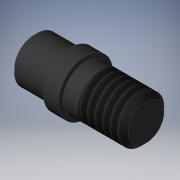
# Autodesk Inventor part: NTBG6-4_a
Saved by Autodesk Inventor 2019 (Build 230136000, 136)
## iProperties
Created: 2023-12-09
Part Number: NTBG6-4_a
Material: Generic
Catalog Web Link: www.cadenas.de
Description: NTBG, NTSBG, NTBGT, NTSBGT_a-Bearings with Male Threads
Vendor: MISUMI
Document SubType Name: Modeling
Designer: psAdmin
Manufacturer: MISUMI
Mass: 0.0517918 g
Surface Area: 0.971102 cm^2
Volume: 0.0517918 cm^3
Density: 1 g/cm^3
Appearance: PSOLRGB-175-175-175
Category: PARTsolutions
Company: MISUMI
Title: NTBG6-4
Author: Cadenas PARTsolutions
Comments: Bearings with Male Threads
PSOL_IDENT_0: {$CADENAS_DATA/23d-libs/misumi/metric/53_rollers/ntbg.prj},185 {VTYP=3D},{NB=NTBG6-4_a},{LINA=NTBG6-
PSOL_IDENT_1: 4},{NN=NTBG, NTSBG, NTBGT, NTSBGT_a},{DATE=09.02.2023 08:01:19},{GEOMDATE=03.02.2023 06:00:02},{VERS
PSOL_IDENT_2: ION=},{LINEID=10},{WBVAR=TS,MATB},{WBNUMERIC=}  {NB=NTBG6-4_a},{LINA=NTBG6-4},{KT=DUMMY},{PN=NTBG6-4
PSOL_IDENT_3: },{TYPE=NTBG},{TS=},{TSALG= '','Standard Male Thread','T','Long Male Thread' },{MATB=},{MATS=SUJ2},{
PSOL_IDENT_4: ST=Electroless Nickel Plating},{D=6},{L=4},{B=2.5},{DD=3},{AA=1.0},{G=1.5},{M=M3},{M1=3},{BE=673ZZ},
PSOL_IDENT_5: {LSM=4},{LLM=6},{D1=3.6},{B1=2.4200},{G1=1.5},{DIA=0.080},{PITCH=0.5},{Z=0.2}
NB: NTBG6-4_a
NN: NTBG, NTSBG, NTBGT, NTSBGT_a
NT: Bearings with Male Threads
NBSYN: $PN._a
LINA: NTBG6-4
CATALOG: Misumi
PN: NTBG6-4
TS: Standard Male Thread
MATB: Steel
ST: Electroless Nickel Plating
D: 6
L: 4
B: 2.5
DD: 3
AA: 1
G: 1.5
M: M3
BE: 673ZZ
SUPPLIER: MISUMI
ARTICLENO: NTBG6-4_a
BOMINFO: NTBG6-4
CREATOR: CADENAS GmbH
Autodesk Inventor part; units mm, degrees
sketch "Sketch_1" plane through (0, 0, 0) normal (0, 0, 1) x (1, 0, 0)
  line L0 (1, 0) -> (-2.42, 0)
  line L1 (-2.42, 0) -> (-2.42, 1.3)
  line L2 (-2.42, 1.3) -> (-2.22, 1.5)
  line L3 (-2.22, 1.5) -> (-0.04, 1.5)
  arc A0 (-0.04, 1.5) -> (0, 1.54) centre (-0.04, 1.54) ccw
  line L4 (0, 1.54) -> (0, 1.8)
  line L5 (0, 1.8) -> (1, 1.8)
  line L6 (1, 1.8) -> (1, 0)
  line L7 (1, 0) -> (-2.42, 0)
  constraints: 16 end point, 2 point on circle, 1 centre point
revolve "Revolution1" add sketch "Sketch_1" angle 360 about axis through (1, 0, 0) along (1, 0, 0)
sketch "Sketch_5" plane through (0, 0, 0) normal (0, 0, 1) x (1, 0, 0)
  line L0 (5, 0) -> (1, 0)
  line L1 (1, 0) -> (1, 1.5)
  line L2 (1, 1.5) -> (4.6935, 1.5)
  line L3 (4.6935, 1.5) -> (5, 1.1935)
  line L4 (5, 1.1935) -> (5, 0)
  line L5 (5, 0) -> (1, 0)
  constraints: 12 end point
revolve "Revolution2" add sketch "Sketch_5" angle 360 about axis through (5, 0, 0) along (1, 0, 0)
thread "Thread1" size "M3x0.5" class "6g" standard "ISO Metric profile" length 2.6935
sketch "Sketch_2" plane through (-2.42, 0, 0) normal (1, 0, 0) x (0, 0, -1)
  line L0 (-0.75, -0.433) -> (0, -0.866)
  line L1 (0, -0.866) -> (0.75, -0.433)
  line L2 (0.75, -0.433) -> (0.75, 0.433)
  line L3 (0.75, 0.433) -> (0, 0.866)
  line L4 (0, 0.866) -> (-0.75, 0.433)
  line L5 (-0.75, 0.433) -> (-0.75, -0.433)
  constraints: 12 end point
extrude "Extrusion1" cut sketch "Sketch_2" along normal blind 1.5
sketch "Sketch_3" plane through (0, 0, 0) normal (0, 0, 1) x (1, 0, 0)
  line L0 (-0.487, 0) -> (-0.92, 0)
  line L1 (-0.92, 0) -> (-0.92, 0.75)
  line L2 (-0.92, 0.75) -> (-0.487, 0)
  line L3 (-0.487, 0) -> (-0.92, 0)
  constraints: 8 end point
revolve "Revolution3" cut sketch "Sketch_3" angle 360 about axis through (-0.487, 0, 0) along (1, 0, 0)
ref_plane "shaft_to_bearing_XY" through (0, 0, 0) normal (1, 0, 0) x (0, 0, -1)
ref_plane "shaft_to_bearing_YZ" through (0, 0, 0) normal (0, 0, -1) x (0, 1, 0)
ref_plane "shaft_to_bearing_ZX" through (0, 0, 0) normal (0, 1, 0) x (1, 0, 0)
body "Solid1"
